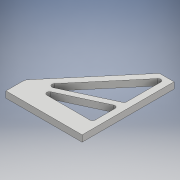
# Autodesk Inventor part: spoilerMount
Saved by Autodesk Inventor 2018.3 (Build 223284000, 284)
## iProperties
Created: 2018-06-23
Part Number: spoilerMount
Material: Generic
Document SubType Name: Modeling
Designer: mzhang
Density: 1 g/cm^3
Appearance: Default
Author: mzhang
Autodesk Inventor part; units mm, degrees
ref_plane "YZ Plane" through (0, 0, 0) normal (1, 0, 0) x (0, 1, 0)
ref_plane "XZ Plane" through (0, 0, 0) normal (0, 1, 0) x (-1, 0, 0)
ref_plane "XY Plane" through (0, 0, 0) normal (0, 0, 1) x (1, 0, 0)
sketch "Sketch1" plane through (0, 0, 0) normal (0, 0, 1) x (1, 0, 0)
  line L0 (0, 0) -> (60, 0)
  line L1 (60, 0) -> (60, 15)
  line L2 (60, 15) -> (0, 15)
  line L3 (0, 13.1718) -> (0, 0)
  line L4 (1.1793, 16.397) -> (51.1793, 75.6283)
  line L5 (60, 72.403) -> (60, 15)
  arc A0 (1.1793, 16.397) -> (0, 13.1718) centre (5, 13.1718) ccw
  arc A1 (60, 72.403) -> (51.1793, 75.6283) centre (55, 72.403) ccw
  dimension "d0" = 60
  dimension "d1" = 15
  dimension "d2" = 5
  constraints: 12 end point, 4 point on circle, 4 tangent, 2 centre point, 2 parallel, 2 point on line, 1 collinear, 1 equal radius, 1 horizontal, 1 perpendicular
  measures "d0" distance of L2.end L1.end
  measures "d1" distance of L1.end L0.end
  measures "d2" radius of A0
extrude "Extrusion1" add sketch "Sketch1" along normal blind 5
sketch "Sketch2" plane through (0, 0, 5) normal (0, 0, 1) x (1, 0, 0)
  arc A0 (1.1793, 16.397) -> (0, 13.1718) centre (5, 13.1718) ccw projected
  arc A1 (60, 72.403) -> (51.1793, 75.6283) centre (55, 72.403) ccw projected
  line L0 (5, 13.1718) -> (55, 72.403)
  line L1 (55, 72.403) -> (55, 13.1718)
  line L2 (55, 13.1718) -> (5, 13.1718)
  line L3 (10, 13.1718) -> (55, 34.0747)
  line L4 (8.2252, 16.9925) -> (55, 38.7198)
  point P0 (0, 0)
  constraints: 10 end point, 4 point on line, 1 parallel, 1 perpendicular, 1 vertical
extrude "Extrusion2" cut sketch "Sketch2" against normal up to surface (5 mm away) contours L0 L1 L4 | L3 L1 L2
fillet "Fillet1" radius 2 6 edges at (8.2252, 16.9925, 2.5) (10, 13.1718, 2.5) (55, 13.1718, 2.5) (55, 34.0747, 2.5) (55, 38.7198, 2.5) (55, 72.403, 2.5)
sketch "Sketch3" plane through (0, 0, 0) normal (0, 0, -1) x (-1, 0, 0)
  line L0 (-100.5339, 103.0883) -> (-24.3212, 103.0883)
  line L1 (-24.3212, 103.0883) -> (-24.3212, 72.403)
  line L2 (-24.3212, 72.403) -> (-100.5339, 72.403)
  line L3 (-100.5339, 72.403) -> (-100.5339, 103.0883)
  point P0 (0, 0)
  constraints: 8 end point, 2 parallel, 1 horizontal, 1 perpendicular
extrude "Extrusion3" cut sketch "Sketch3" against normal up to surface (5 mm away)
sketch "Sketch4" plane through (48.4567, 72.403, 0) normal (0, 1, 0) x (1, 0, 0)
  line L0 (5.3859, 0) -> (5.3859, -5) projected
  circle A0 centre (5.3859, -2.5) radius 1.5
  point P0 (-48.4567, 0)
  dimension "d10" = 3
  constraints: 1 centre point, 1 midpoint
  measures "d10" diameter of A0
extrude "Extrusion4" cut sketch "Sketch4" against normal blind 5
body "Solid1"
